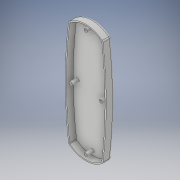
# Autodesk Inventor part: armrest
Saved by Autodesk Inventor 2019.3 (Build 233278000, 278)
## iProperties
Created: 2020-09-17
Part Number: armrest
Material: Generisch
Document SubType Name: Modeling
Designer: Nicolas Frick
Density: 1 g/cm^3
Appearance: Vorgabe
Author: Nicolas Frick
Autodesk Inventor part; units mm, degrees
ref_plane "YZ Plane" through (0, 0, 0) normal (1, 0, 0) x (0, 1, 0)
ref_plane "XZ Plane" through (0, 0, 0) normal (0, 1, 0) x (-1, 0, 0)
ref_plane "XY Plane" through (0, 0, 0) normal (0, 0, 1) x (1, 0, 0)
sketch "Skizze1" plane through (0, 0, 0) normal (0, 0, 1) x (1, 0, 0)
  line L0 (0, 0) -> (56.5, 0) construction
  line L1 (56.5, 0) -> (56.5, -183.5) construction
  line L2 (0, 0) -> (56.5, 0) construction
  line L3 (56.5, 0) -> (56.5, -183.5) construction
  line L4 (56.5, -183.5) -> (0, -183.5) construction
  line L5 (0, -183.5) -> (0, 0) construction
  line L6 (28.25, 0) -> (28.25, 3) construction
  line L7 (28.25, -183.5) -> (28.25, -186.5) construction
  line L8 (28.25, -91.75) -> (1.75, -91.75) construction
  line L9 (28.25, -91.75) -> (-5.75, -91.75) construction
  line L10 (28.25, -91.75) -> (54.75, -91.75) construction
  line L11 (28.25, -91.75) -> (62.25, -91.75) construction
  circle A0 centre (28.25, 3) radius 1.5
  circle A1 centre (28.25, 3) radius 3
  line L12 (28.25, 3) -> (28.25, 10.5) construction
  circle A2 centre (28.25, -186.5) radius 1.5
  circle A3 centre (28.25, -186.5) radius 3
  line L13 (28.25, -186.5) -> (28.25, -194) construction
  circle A4 centre (1.75, -91.75) radius 1.5
  circle A5 centre (1.75, -91.75) radius 3
  circle A6 centre (54.75, -91.75) radius 1.5
  circle A7 centre (54.75, -91.75) radius 3
  line L14 (28.25, -183.5) -> (28.25, -153.093) construction
  line L15 (0, 0) -> (-5.75, -91.75) construction
  line L16 (-5.75, -91.75) -> (0, -183.5) construction
  line L17 (62.25, -91.75) -> (56.25, 0) construction
  arc A8 (0, 0) -> (0, -183.5) centre (729.1304, -91.75) ccw
  line L18 (60.0727, -126.4918) -> (62.25, -91.75) construction
  arc A9 (56.5, 0) -> (0, 0) centre (28.25, -32.753) ccw
  arc A10 (56.5, -183.5) -> (56.5, 0) centre (-672.6304, -91.75) ccw
  arc A11 (0, -183.5) -> (56.5, -183.5) centre (28.25, -150.747) ccw
  constraints: 38 end point, 12 centre point, 12 coincident, 12 point on circle, 5 horizontal, 4 vertical, 3 parallel, 3 perpendicular, 2 midpoint, 2 point on line
extrude "Extrusion1" add sketch "Skizze1" along normal blind 3 contours A9 A10 A11 A8
sketch "Skizze2" plane through (0, 0, 0) normal (0, 0, -1) x (-1, 0, 0)
  circle A0 centre (-54.75, -91.75) radius 3 construction
  circle A1 centre (-1.75, -91.75) radius 3 construction
  circle A2 centre (-28.25, -186.5) radius 3 construction
  circle A3 centre (-28.25, 3) radius 3 construction
  arc A4 (0, -183.5) -> (0, 0) centre (-729.1304, -91.75) ccw projected
  arc A5 (0, 0) -> (-56.5, 0) centre (-28.25, -32.753) ccw projected
  arc A6 (-56.5, 0) -> (-56.5, -183.5) centre (672.6304, -91.75) ccw projected
  arc A7 (-56.5, -183.5) -> (0, -183.5) centre (-28.25, -150.747) ccw projected
  arc A8 (1.8892, -184.5029) -> (1.8892, 1.0029) centre (-729.1304, -91.75) ccw
  arc A9 (-58.3892, -184.5029) -> (1.8892, -184.5029) centre (-28.25, -150.747) ccw
  arc A10 (-58.3892, 1.0029) -> (-58.3892, -184.5029) centre (672.6304, -91.75) ccw
  arc A11 (1.8892, 1.0029) -> (-58.3892, 1.0029) centre (-28.25, -32.753) ccw
  dimension "d25" = 2
  constraints: 8 point on circle, 4 centre point, 3 other
  measures "d25" radial gap between concentric circles of A4 A8
extrude "Extrusion2" add sketch "Skizze2" against normal blind 15
sketch "Skizze3" plane through (0, 0, 0) normal (0, 0, -1) x (-1, 0, 0)
  circle A0 centre (-28.25, 3) radius 3 projected
  circle A1 centre (-1.75, -91.75) radius 3 projected
  circle A2 centre (-54.75, -91.75) radius 3 projected
  circle A3 centre (-28.25, -186.5) radius 3 projected
  point P0 (0, 0)
extrude "Extrusion3" add sketch "Skizze3" against normal blind 15
sketch "Skizze4" plane through (28.25, 3, 15) normal (0, 0, 1) x (1, 0, 0)
  circle A0 centre (0, 0) radius 1.5
  circle A1 centre (-26.5, -94.75) radius 3 construction
  circle A2 centre (26.5, -94.75) radius 3 construction
  circle A3 centre (0, -189.5) radius 3 construction
  circle A4 centre (-26.5, -94.75) radius 1.5
  circle A5 centre (26.5, -94.75) radius 1.5
  circle A6 centre (0, -189.5) radius 1.5
  point P0 (-28.25, -3)
  dimension "d30" = 3
  dimension "d31" = 3
  dimension "d32" = 3
  dimension "d33" = 3
  constraints: 4 centre point, 3 coincident
  measures "d30" diameter of A0
  measures "d31" diameter of A4
  measures "d32" diameter of A5
  measures "d33" diameter of A6
extrude "Extrusion4" cut sketch "Skizze4" against normal blind 10
fillet "Rundung1" radius 2 4 edges at (0, 0, 9) (56.5, 0, 9) (56.5, -183.5, 9) (0, -183.5, 9)
fillet "Rundung2" radius 4 8 edges at (64.25, -91.75, 0) (58.3892, 1.0029, 7.5) (28.25, 12.5, 0) (28.25, -196, 0) (-7.75, -91.75, 0) (-1.8892, 1.0029, 7.5) (58.3892, -184.5029, 7.5) (-1.8892, -184.5029, 7.5)
